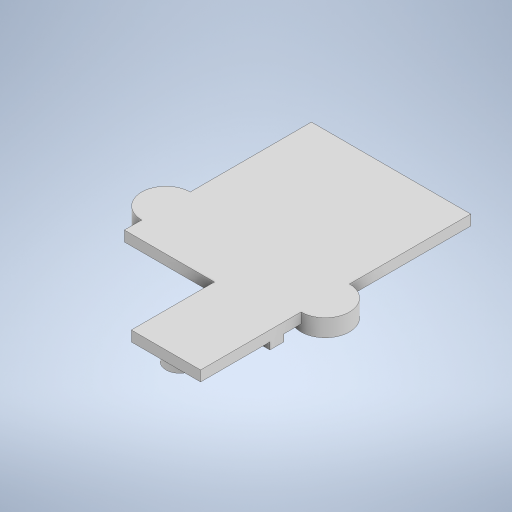
# Autodesk Inventor part: type_A_ver2
Saved by Autodesk Inventor 2024.1 (Build 281209000, 209)
## iProperties
Created: 2025-04-13
Part Number: type_A_ver2
Material: 一般
Document SubType Name: Modeling
Designer: hibik
Density: 1 g/cm^3
Appearance: 既定
Author: hibik
Autodesk Inventor part; units mm, degrees
ref_plane "YZ Plane" through (0, 0, 0) normal (1, 0, 0) x (0, 1, 0)
ref_plane "XZ Plane" through (0, 0, 0) normal (0, 1, 0) x (-1, 0, 0)
ref_plane "XY Plane" through (0, 0, 0) normal (0, 0, 1) x (1, 0, 0)
sketch "スケッチ1" plane through (0, 0, 0) normal (0, 1, 0) x (-1, 0, 0)
  line L0 (0, 0) -> (30, 0)
  line L1 (30, 0) -> (30, -27)
  line L2 (30, -27) -> (0, -27)
  line L3 (0, -27) -> (0, 0)
  circle A0 centre (26.5, -6) radius 3.5
  circle A1 centre (3.5, -6) radius 3.5
  line L4 (26.5, 0) -> (26.5, -27)
  line L5 (3.5, -27) -> (3.5, 0)
  point P0 (26.5, -9.5)
  point P1 (26.5, -2.5)
  point P2 (3.5, -2.5)
  point P3 (3.5, -9.5)
  dimension "d0" = 30
  dimension "d1" = 27
  dimension "d2" = 7
  dimension "d3" = 7
  dimension "d4" = 6
  constraints: 12 end point, 6 point on line, 2 centre point, 2 parallel, 2 perpendicular, 2 tangent, 1 horizontal, 1 horizontal alignment, 1 vertical
  measures "d0" distance of L1.end L2.end
  measures "d1" distance of L0.end L1.end
  measures "d2" diameter of A0
  measures "d3" diameter of A1
  measures "d4" distance from line of L0 A0.centre
extrude "押し出し1" add sketch "スケッチ1" along normal blind 1.5 contours L0 L4 A0 L2 L5 A1 | A1 L5 | A1 L5 | L4 A0 | A0 L4
sketch "スケッチ2" plane through (0, 1.5, 0) normal (0, 1, 0) x (1, 0, 0)
  line L0 (-3.5, 0) -> (-13.5, 0)
  line L1 (-13.5, 0) -> (-13.5, -12)
  line L2 (-13.5, -12) -> (-3.5, -12)
  line L3 (-3.5, -12) -> (-3.5, 0)
  line L4 (-3.5, 0) -> (-3.5, 2.5) projected
  point P0 (0, 0)
  dimension "d7" = 10
  dimension "d8" = 12
  constraints: 8 end point, 2 parallel, 1 horizontal, 1 perpendicular
  measures "d7" distance of L2.end L1.end
  measures "d8" distance of L1.end L0.end
extrude "押し出し2" add sketch "スケッチ2" against normal up to surface (1.5 mm away)
sketch "スケッチ3" plane through (0, 0, 0) normal (0, -1, 0) x (1, 0, 0)
  arc A0 (-26.5, -2.5) -> (-26.5, -9.5) centre (-26.5, -6) ccw projected
  arc A1 (-3.5, -9.5) -> (-3.5, -2.5) centre (-3.5, -6) ccw projected
  line L0 (-26.5, 0) -> (-13.5, 0) projected
  line L1 (-13.5, 0) -> (-3.5, 0)
  line L2 (-3.5, 0) -> (-3.5, 2)
  line L3 (-3.5, 2) -> (-13.5, 2)
  line L4 (-13.5, 2) -> (-13.5, 0)
  line L5 (-3.5, -2.5) -> (-3.5, 12) projected
  circle A2 centre (-26.5, -6) radius 3.5
  circle A3 centre (-3.5, -6) radius 3.5
  point P0 (0, 0)
  point P1 (-3.5, -2.5)
  point P2 (-26.5, -9.5)
  dimension "d11" = 2
  constraints: 8 end point, 2 centre point, 2 coincident, 2 concentric, 2 parallel, 1 collinear, 1 horizontal, 1 perpendicular
  measures "d11" distance of L1.end L2.end
extrude "押し出し3" add sketch "スケッチ3" along normal blind 1
sketch "スケッチ4" plane through (0, 0, 0) normal (0, -1, 0) x (1, 0, 0)
  circle A0 centre (-8.5, 10) radius 2
  line L0 (-3.5, 12) -> (-13.5, 12) projected
  point P0 (0, 0)
  point P1 (-8.5, 12)
  dimension "d14" = 4
  constraints: 1 centre point, 1 midpoint, 1 tangent, 1 vertical alignment
  measures "d14" diameter of A0
extrude "押し出し4" add sketch "スケッチ4" along normal blind 1
